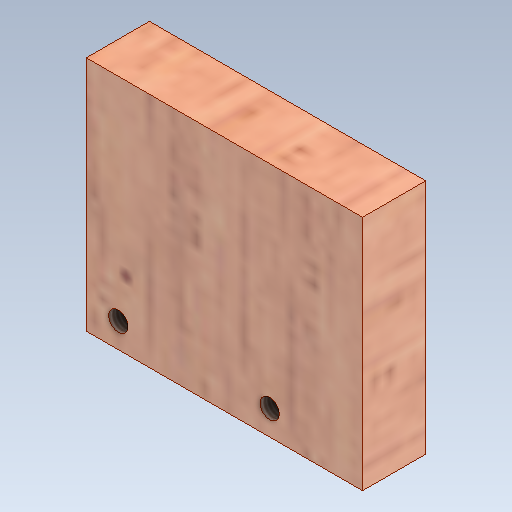
# Autodesk Inventor part: 0005-10-028 suport senzor y
Saved by Autodesk Inventor 2020 (Build 240168000, 168)
## iProperties
Created: 2020-12-18
Part Number: 0005-10-028 suport senzor y
Material: Generic
Document SubType Name: Modeling
Designer: Iulian Bors
Density: 1 g/cm^3
Appearance: White Oak - Natural Medium Gloss
Mass: 7.40606 g
Surface Area: 35.4744 cm^2
Volume: 7.40606 cm^3
Author: Iulian Bors
Subject: 028
Autodesk Inventor part; units mm, degrees
ref_plane "YZ Plane" through (0, 0, 0) normal (1, 0, 0) x (0, 1, 0)
ref_plane "XZ Plane" through (0, 0, 0) normal (0, 1, 0) x (-1, 0, 0)
ref_plane "XY Plane" through (0, 0, 0) normal (0, 0, 1) x (1, 0, 0)
sketch "Sketch1" plane through (0, 0, 0) normal (0, 0, 1) x (1, 0, 0)
  line L0 (-17.5, 15) -> (17.5, 15)
  line L1 (17.5, 15) -> (17.5, -15)
  line L2 (17.5, -15) -> (-17.5, -15)
  line L3 (-17.5, -15) -> (-17.5, 15)
  point P0 (0, 0)
  point P1 (0, 15)
  point P2 (-17.5, 0)
  dimension "d0" = 35
  dimension "d1" = 30
  constraints: 8 end point, 2 midpoint, 2 parallel, 1 horizontal, 1 horizontal alignment, 1 perpendicular, 1 vertical alignment
  measures "d0" distance of L0.start L0.end
  measures "d1" distance of L2.end L0.start
extrude "Extrusion1" add sketch "Sketch1" along normal blind 8
sketch "Sketch6" plane through (0, 0, 8) normal (0, 0, 1) x (1, 0, 0)
  circle A0 centre (5.7312, -11.8725) radius 1.7875 projected
  circle A1 centre (-13.4438, -11.8725) radius 1.7875 projected
  point P0 (0, 0)
hole "Hole1" at (5.7312, -11.8725, 8) at (-13.4438, -11.8725, 8) direction (0, 0, -1) diameter 2.459 end through all thread size "M3x0.5" class "6H" standard "ISO Metric profile"
body "Solid1"
